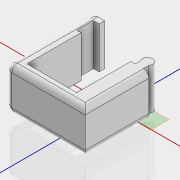
# Autodesk Inventor part: ЛЦМК.30000.10.00.03 Крышка передняя
Saved by Autodesk Inventor 2021.2 (Build 252289000, 289)
## iProperties
Created: 2025-11-22
Part Number: ЛЦМК.30000.10.00.03 Крышка передняя
Material: Типовые
Document SubType Name: Modeling
Designer: Захаров
Density: 1 g/cm^3
Appearance: По умолчанию
Author: Захаров
Autodesk Inventor part; units mm, degrees
ref_plane "YZ Plane" through (0, 0, 0) normal (1, 0, 0) x (0, 1, 0)
ref_plane "XZ Plane" through (0, 0, 0) normal (0, 1, 0) x (-1, 0, 0)
ref_plane "XY Plane" through (0, 0, 0) normal (0, 0, 1) x (1, 0, 0)
ref_plane "РабПлоскость1" through (-0.858, 10.5846, 17.8317) normal (0, -1, 0) x (1, 0, 0)
ref_plane "РабПлоскость2" through (4.892, 13.1846, 45.3317) normal (0, 1, 0) x (1, 0, 0)
sketch "Эскиз1" plane through (-0.858, 13.1846, 17.8317) normal (0, -1, 0) x (1, 0, 0)
  arc A0 (8.858, -19.8317) -> (11.858, -19.8317) centre (10.358, -20.8267) ccw projected
  line L0 (8.858, -19.8317) -> (8.858, -17.8317) projected
  line L1 (11.858, -17.8317) -> (11.858, -19.8317) projected
  line L2 (11.958, -17.8317) -> (11.958, -21.4012)
  arc A1 (8.958, -21.7911) -> (11.958, -21.4012) centre (10.358, -20.8267) ccw
  line L3 (8.958, -21.7911) -> (8.958, -17.8317)
  line L4 (11.858, -17.8317) -> (13.858, -17.8317) projected
  line L5 (4.858, -17.8317) -> (8.858, -17.8317) projected
  line L6 (7.358, -19.8317) -> (7.358, 1.6683) projected
  line L7 (7.358, 1.6683) -> (-10.642, 1.6683) projected
  line L8 (-10.642, 1.6683) -> (-10.642, -19.8317) projected
  line L9 (-12.142, -17.8317) -> (-8.142, -17.8317) projected
  line L10 (-12.142, -23.8317) -> (-12.142, -17.8317) projected
  line L11 (13.858, -17.8317) -> (13.858, 5.1683)
  line L12 (13.858, 5.1683) -> (-14.5723, 5.1683)
  line L13 (-14.5723, 5.1683) -> (-14.5723, -25.8317)
  line L14 (-14.5723, -25.8317) -> (-10.142, -25.8317)
  line L15 (-10.142, -25.8317) -> (-10.142, -23.8317)
  line L16 (-12.142, -23.8317) -> (-10.142, -23.8317)
  line L17 (8.858, -17.8317) -> (8.958, -17.8317)
  line L18 (11.858, -17.8317) -> (11.958, -17.8317)
  point P0 (0.858, -17.8317)
  point P1 (-10.642, -17.8317)
  point P2 (7.358, -17.8317)
  point P3 (19.5, 6.5781)
  point P4 (19.5, 4.3408)
  point P5 (1.1058, 1.6683)
  point P6 (19.1666, -17.8317)
  point P7 (11.858, -18.4138)
  point P8 (-4.2637, -11.6345)
  point P9 (-4.2637, 1.6683)
  dimension "d0" = 0.1
  dimension "d1" = 23
  dimension "d2" = 2
  dimension "d3" = 2
  constraints: 20 end point, 5 perpendicular, 2 point on circle, 1 centre point, 1 collinear, 1 horizontal, 1 vertical, 2 other
  measures "d0" radial gap between concentric circles of A0 A1
  measures "d1" distance of L4.end L11.end
  measures "d2" vertical distance of L13.end L10.start
  measures "d3" horizontal distance of L14.end L10.start
extrude "Выдавливание1" add sketch "Эскиз1" against normal blind 15 contours L0 L17 L3 A1 L2 A0 | L2 A1 L3 L17 L5 L6 L7 L8 L9 L10 L16 L15 L14 L13 L12 L11 L4 L1 A0
fillet "Сопряжение1" radius 2 8 edges at (-15.4303, 20.6846, -8) (-15.4303, 13.1846, 7.5) (-15.4303, 28.1846, 7.5) (-15.4303, 20.6846, 23) (-1.2151, 13.1846, 23) (-1.2151, 28.1846, 23) (13, 13.1846, 11.5) (13, 28.1846, 11.5)
